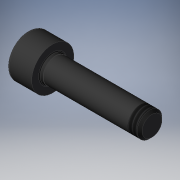
# Autodesk Inventor part: Slotted head cap screw ISO 4762 - M5x20
Saved by Autodesk Inventor 2024 (Build 280153000, 153)
## iProperties
Created: 2023-06-23
Part Number: Slotted head cap screw ISO 4762 - M5x20
Material: Generic
Catalog Web Link: www.cadenas.de
Description: ISO 4762-Hexagon socket head cap screw
Vendor: MISUMI
Document SubType Name: Modeling
Designer: psAdmin
Manufacturer: MISUMI
Mass: 0.626495 g
Surface Area: 5.92343 cm^2
Volume: 0.626495 cm^3
Density: 1 g/cm^3
Appearance: PSOLRGB-175-175-175
Category: PARTsolutions
Company: MISUMI
PSOL_IDENT_0: {$CADENAS_DATA/23d-libs/misumi/metric/accessories/din_en_iso_4762.prj},221 {VTYP=3D},{NB=Slotted hea
PSOL_IDENT_1: d cap screw ISO 4762 - M5x20},{LINA=Slotted head cap screw ISO 4762 - M5x20},{NN=ISO 4762},{DATE=13.
PSOL_IDENT_2: 07.2021 11:48:40},{GEOMDATE=21.06.2021 06:17:40},{VERSION=},{LINEID=510},{WBVAR=},{WBNUMERIC=}  {NB=
PSOL_IDENT_3: Zylinderschraube ISO 4762 - M5x20},{LINA=Zylinderschraube ISO 4762 - M5x20},{KT=DUMMY},{IDNR=},{D=5.
PSOL_IDENT_4: 000},{D3=4.019},{P=0.800},{L=20.000},{S=4.000},{HM=20.000},{DK=8.500},{DA=5.700},{DS=5.000},{E=4.580
PSOL_IDENT_5: },{K=5.000},{R=0.200},{T=2.500},{V=0.500},{DW=8.030},{W=1.900},{LF=0.600},{LG=2.400},{FORM=1.000},{N
PSOL_IDENT_6: ENN=M5x20}
NB: Slotted head cap screw ISO 4762 - M5x20
NN: ISO 4762
NT: Hexagon socket head cap screw
NBSYN: Slotted head cap screw ISO 4762 - $NENN.
LINA: Slotted head cap screw ISO 4762 - M5x20
CATALOG: Misumi
ROWDESC: M5x20
D: 5
D3: 4.019
P: 0.8
L: 20
S: 4
HM: 20
DK: 8.5
DA: 5.7
DS: 5
E: 4.58
K: 5
R: 0.2
T: 2.5
V: 0.5
DW: 8.03
W: 1.9
LF: 0.6
LG: 2.4
FORM: 1
SUPPLIER: MISUMI
ARTICLENO: Slotted head cap screw ISO 4762 - M5x20
BOMINFO: Slotted head cap screw ISO 4762 - M5x20
CREATOR: CADENAS GmbH
Title: Slotted head cap screw ISO 4762 - M5x20
Author: Cadenas PARTsolutions
Comments: Hexagon socket head cap screw
Autodesk Inventor part; units mm, degrees
sketch "Skizze_2" plane through (0, 0, 0) normal (0, 0, 1) x (1, 0, 0)
  line L0 (20, 0) -> (-0.7453, 0)
  line L1 (-0.7453, 0) -> (-1.9, 2)
  line L2 (-1.9, 2) -> (-5, 2)
  line L3 (-5, 2) -> (-5, 3.75)
  arc A0 (-4.5, 4.25) -> (-5, 3.75) centre (-4.5, 3.75) ccw
  line L4 (-4.5, 4.25) -> (0, 4.25)
  line L5 (0, 4.25) -> (0, 2.85)
  arc A1 (0, 2.85) -> (0.1298, 2.6627) centre (0.2, 2.85) ccw
  line L6 (0.1298, 2.6627) -> (0.5298, 2.5127)
  arc A2 (0.5298, 2.5127) -> (0.6, 2.5) centre (0.6, 2.7) ccw
  line L7 (0.6, 2.5) -> (19.5095, 2.5)
  line L8 (19.5095, 2.5) -> (20, 2.0095)
  line L9 (20, 2.0095) -> (20, 0)
  line L10 (20, 0) -> (-0.7453, 0)
  constraints: 22 end point, 6 point on circle, 3 centre point
revolve "Revolution1" add sketch "Skizze_2" angle 360 about axis through (20, 0, 0) along (1, 0, 0)
thread "Thread1" size "M5x0.8" class "6g" standard "ISO Metric profile" length 1.9095
sketch "Skizze_1" plane through (-1.9, 0, 0) normal (1, 0, 0) x (0, 0, -1)
  line L0 (-2, -1.1547) -> (0, -2.3094)
  line L1 (0, -2.3094) -> (2, -1.1547)
  line L2 (2, -1.1547) -> (2, 1.1547)
  line L3 (2, 1.1547) -> (0, 2.3094)
  line L4 (0, 2.3094) -> (-2, 1.1547)
  line L5 (-2, 1.1547) -> (-2, -1.1547)
  constraints: 12 end point
extrude "Extrusion1" cut sketch "Skizze_1" against normal blind 5
ref_plane "IP1_XY" through (0, 0, 0) normal (1, 0, 0) x (0, 0, -1)
ref_plane "IP1_YZ" through (0, 0, 0) normal (0, 0, -1) x (0, 1, 0)
ref_plane "IP1_ZX" through (0, 0, 0) normal (0, 1, 0) x (1, 0, 0)
ref_plane "IP2_XY" through (-5, 0, 0) normal (1, 0, 0) x (0, 0, -1)
ref_plane "IP2_YZ" through (-5, 0, 0) normal (0, 0, -1) x (0, 1, 0)
ref_plane "IP2_ZX" through (-5, 0, 0) normal (0, 1, 0) x (1, 0, 0)
ref_plane "IP3_XY" through (20, 0, 0) normal (1, 0, 0) x (0, 0, -1)
ref_plane "IP3_YZ" through (20, 0, 0) normal (0, 0, -1) x (0, 1, 0)
ref_plane "IP3_ZX" through (20, 0, 0) normal (0, 1, 0) x (1, 0, 0)
ref_plane "IP4_XY" through (0, 0, 0) normal (1, 0, 0) x (0, 0, -1)
ref_plane "IP4_YZ" through (0, 0, 0) normal (0, 0, -1) x (0, 1, 0)
ref_plane "IP4_ZX" through (0, 0, 0) normal (0, 1, 0) x (1, 0, 0)
body "Solid1"
